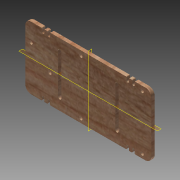
# Autodesk Inventor part: electronics_pouch
Saved by Autodesk Inventor 2015 (Build 190159000, 159)
## iProperties
Created: 2014-11-09
Part Number: electronics_pouch
Material: Wood (Birch)
Document SubType Name: Modeling
Designer: rawrdong
Density: 0.55 g/cm^3
Appearance: Birch - Natural Polished
Author: rawrdong
Autodesk Inventor part; units mm, degrees
ref_plane "YZ Plane" through (0, 0, 0) normal (1, 0, 0) x (0, 1, 0)
ref_plane "XZ Plane" through (0, 0, 0) normal (0, 1, 0) x (-1, 0, 0)
ref_plane "XY Plane" through (0, 0, 0) normal (0, 0, 1) x (1, 0, 0)
sketch "Sketch1" plane through (0, 0, 0) normal (0, 1, 0) x (-1, 0, 0)
  line L0 (0, 0) -> (110, 0)
  line L1 (110, 0) -> (110, -55)
  line L2 (110, -55) -> (0, -55)
  line L3 (0, -55) -> (0, 0)
  line L4 (55, 0) -> (55, -55) construction
  circle A0 centre (8, -4.1151) radius 1.425
  circle A1 centre (8, -51.4351) radius 1.425
  circle A2 centre (61.47, -4.1151) radius 1.425
  circle A3 centre (61.47, -51.4351) radius 1.425
  line L5 (8, -4.1151) -> (61.47, -4.1151) construction
  line L6 (61.47, -4.1151) -> (61.47, -51.4351) construction
  line L7 (61.47, -51.4351) -> (8, -51.4351) construction
  line L8 (8, -51.4351) -> (8, -4.1151) construction
  line L9 (80, -10) -> (80, -45) construction
  line L10 (78.575, -10) -> (78.575, -45)
  line L11 (81.425, -45) -> (81.425, -10)
  arc A4 (81.425, -10) -> (78.575, -10) centre (80, -10) ccw
  arc A5 (78.575, -45) -> (81.425, -45) centre (80, -45) ccw
  line L12 (30, -10) -> (30, -45) construction
  line L13 (28.575, -10) -> (28.575, -45)
  line L14 (31.425, -45) -> (31.425, -10)
  arc A6 (31.425, -10) -> (28.575, -10) centre (30, -10) ccw
  arc A7 (28.575, -45) -> (31.425, -45) centre (30, -45) ccw
  circle A8 centre (105.075, -15.8851) radius 1.425
  circle A9 centre (88.565, -30.4901) radius 1.425
  line L15 (108, -12.9601) -> (86.41, -12.9601) construction
  line L16 (86.41, -12.9601) -> (86.41, -43.4401) construction
  line L17 (86.41, -43.4401) -> (108, -43.4401) construction
  line L18 (108, -43.4401) -> (108, -12.9601) construction
  line L19 (105.075, -15.8851) -> (108, -15.8851) construction
  line L20 (105.075, -15.8851) -> (105.075, -12.9601) construction
  point P0 (80, -27.5)
  point P1 (30, -27.5)
  point P2 (55, -27.5)
  dimension "d4" = 53.47
  dimension "d5" = 47.32
  dimension "d12" = 1.425
  dimension "d13" = 50
  dimension "d14" = 2.85
  dimension "d15" = 14.605
  dimension "d16" = 16.51
  dimension "d17" = 21.59
  dimension "d18" = 30.48
  dimension "d19" = 2.925
  dimension "d20" = 8
  dimension "d21" = 2
  dimension "d22" = 55
  dimension "d23" = 110
  dimension "d34" = 35
  constraints: 46 end point, 10 centre point, 9 parallel, 8 point on circle, 8 tangent, 6 equal radius, 5 midpoint, 4 perpendicular, 3 horizontal, 2 coincident, 2 equal length, 2 horizontal alignment, 2 point on line, 2 vertical, 1 other
  measures "d4" distance of L6.end L7.end
  measures "d5" distance of L5.end L6.end
  measures "d12" radius of A6
  measures "d13" distance between parallel lines of L12 L9
  measures "d14" diameter of A2
  measures "d15" vertical distance of A9.centre L19.start
  measures "d16" horizontal distance of A9.centre L19.start
  measures "d17" distance of L15.start L15.end
  measures "d18" distance of L17.end L15.start
  measures "d19" distance from line of L19.start L15
  measures "d20" distance between parallel lines of L3 L8
  measures "d21" distance between parallel lines of L1 L18
  measures "d22" distance of L2.end L0.start
  measures "d23" distance of L1.end L2.end
  measures "d34" distance of L12.start L12.end
extrude "Extrusion1" add sketch "Sketch1" along normal blind 3
fillet "Fillet1" radius 5 4 edges at (0, 1.5, -55) (-110, 1.5, -55) (0, 1.5, 0) (-110, 1.5, 0)
sketch "Sketch2" plane through (0, 0, 0) normal (0, -1, 0) x (1, 0, 0)
  arc A0 (-28.575, -10) -> (-31.425, -10) centre (-30, -10) ccw projected
  line L0 (-28.575, -10) -> (-28.575, -45) projected
  arc A1 (-31.425, -45) -> (-28.575, -45) centre (-30, -45) ccw projected
  line L1 (-31.425, -45) -> (-31.425, -10) projected
  arc A2 (-78.575, -10) -> (-81.425, -10) centre (-80, -10) ccw projected
  line L2 (-78.575, -10) -> (-78.575, -45) projected
  arc A3 (-81.425, -45) -> (-78.575, -45) centre (-80, -45) ccw projected
  line L3 (-81.425, -45) -> (-81.425, -10) projected
  circle A4 centre (-88.565, -30.4901) radius 1.425 projected
  circle A5 centre (-105.075, -15.8851) radius 1.425 projected
  circle A6 centre (-61.47, -51.4351) radius 1.425 projected
  circle A7 centre (-61.47, -4.1151) radius 1.425 projected
  circle A8 centre (-8, -51.4351) radius 1.425 projected
  circle A9 centre (-8, -4.1151) radius 1.425 projected
  arc A10 (-105, 0) -> (-110, -5) centre (-105, -5) ccw projected
  line L4 (-110, -5) -> (-110, -50) projected
  arc A11 (-110, -50) -> (-105, -55) centre (-105, -50) ccw projected
  line L5 (-105, -55) -> (-5, -55) projected
  arc A12 (-5, -55) -> (0, -50) centre (-5, -50) ccw projected
  line L6 (0, -50) -> (0, -5) projected
  arc A13 (0, -5) -> (-5, 0) centre (-5, -5) ccw projected
  line L7 (-5, 0) -> (-105, 0) projected
  line L8 (-105, 0) -> (-5, 0) projected
  circle A14 centre (-20.937, 0) radius 1.5
  line L9 (-5, -55) -> (-105, -55) projected
  line L10 (-55, -55) -> (-55, 0) construction
  line L11 (-110, -50) -> (-110, -5) projected
  line L12 (-110, -27.5) -> (0, -27.5) construction
  circle A15 centre (-15.937, 0) radius 1.5
  circle A16 centre (-89.063, 0) radius 1.5
  circle A17 centre (-94.063, 0) radius 1.5
  circle A18 centre (-20.937, -55) radius 1.5
  circle A19 centre (-15.937, -55) radius 1.5
  circle A20 centre (-89.063, -55) radius 1.5
  circle A21 centre (-94.063, -55) radius 1.5
  point P0 (0, 0)
  dimension "d24" = 3
  dimension "d27" = 5
  constraints: 8 centre point, 6 symmetric about line, 4 end point, 4 midpoint, 2 point on line, 1 equal radius, 6 other
  measures "d24" diameter of A14
  measures "d27" distance of A15.centre A14.centre
extrude "Extrusion2" [suppressed]
sketch "Sketch3" plane through (0, 0, 0) normal (0, -1, 0) x (1, 0, 0)
  line L0 (-5, 0) -> (-105, 0) projected
  line L1 (0, -50) -> (0, -5) projected
  line L2 (-105, -55) -> (-5, -55) projected
  line L3 (-110, -5) -> (-110, -50) projected
  circle A0 centre (-20.551, -3) radius 1
  circle A1 centre (-15.551, -3) radius 1
  line L4 (-21.551, -3) -> (-21.551, 0)
  line L5 (-19.551, -3) -> (-19.551, 0)
  line L6 (-16.551, -3) -> (-16.551, 0)
  line L7 (-14.551, -3) -> (-14.551, 0)
  point P0 (0, 0)
  dimension "d28" = 2
  dimension "d29" = 5
  dimension "d30" = 3
  constraints: 8 end point, 4 point on circle, 4 point on line, 4 tangent, 3 perpendicular, 2 centre point, 1 equal radius, 1 horizontal alignment, 1 vertical
  measures "d28" diameter of A0
  measures "d29" distance of A1.centre A0.centre
  measures "d30" distance of L7.start L7.end
extrude "Extrusion3" cut sketch "Sketch3" against normal through all
ref_plane "Work Plane1" through (-105, 0, -27.5) normal (0, 0, 1) x (1, 0, 0)
ref_plane "Work Plane2" through (-55, 0, -5) normal (1, 0, 0) x (0, 0, -1)
mirror "Mirror1" about plane through (-105, 0, -27.5) normal (0, 0, 1) of "Extrusion3"
mirror "Mirror2" about plane through (-55, 0, -5) normal (1, 0, 0) of "Extrusion3", "Mirror1"
fillet "Fillet2" radius 0.5 16 edges at (-21.551, 1.5, 0) (-19.551, 1.5, 0) (-16.551, 1.5, 0) (-14.551, 1.5, 0) (-14.551, 1.5, -55) (-16.551, 1.5, -55) (-19.551, 1.5, -55) (-21.551, 1.5, -55) (-88.449, 1.5, -55) (-90.449, 1.5, -55) (-93.449, 1.5, -55) (-95.449, 1.5, -55) (-95.449, 1.5, 0) (-93.449, 1.5, 0) (-90.449, 1.5, 0) (-88.449, 1.5, 0)
body "Solid1"
